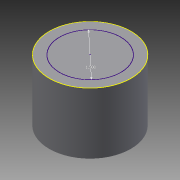
# Autodesk Inventor part: rotating base
Saved by Autodesk Inventor 2014 (Build 180170000, 170)
## iProperties
Created: 2017-01-04
Part Number: rotating base
Material: Generic
Document SubType Name: Modeling
Designer: lloi
Density: 1 g/cm^3
Appearance: Default
Author: lloi
Autodesk Inventor part; units mm, degrees
ref_plane "YZ Plane" through (0, 0, 0) normal (1, 0, 0) x (0, 1, 0)
ref_plane "XZ Plane" through (0, 0, 0) normal (0, 1, 0) x (-1, 0, 0)
ref_plane "XY Plane" through (0, 0, 0) normal (0, 0, 1) x (1, 0, 0)
sketch "Sketch1" plane through (0, 0, 0) normal (0, 1, 0) x (-1, 0, 0)
  circle A0 centre (0, 0) radius 25.4
  dimension "d0" = 50.8
  constraints: 1 centre point, 1 coincident
  measures "d0" diameter of A0
extrude "Extrusion1" add sketch "Sketch1" along normal blind 38.1
sketch "Sketch3" plane through (0, 38.1, 0) normal (0, 1, 0) x (1, 0, 0)
  circle A0 centre (0, 0) radius 25.4 projected
  circle A1 centre (0, 0) radius 19.05
  dimension "d6" = 38.1
  constraints: 1 centre point, 1 coincident
  measures "d6" diameter of A1
body "Solid1"
